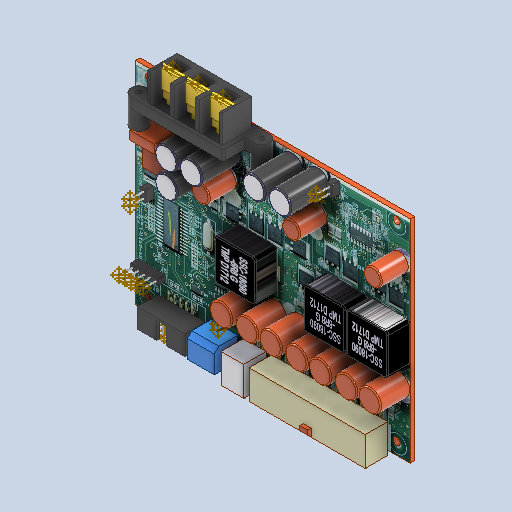
# Autodesk Inventor part: N40L
Saved by Autodesk Inventor 2022 (Build 260153000, 153)
## iProperties
Company: Hitatchi
Created: 2022-10-18
Checked By: Баранчук
Material: Phenolic Resin
Document SubType Name: Modeling
Density: 1.38 g/cm^3
Appearance: Smooth - Light Orange
Categories: <MemberInstance><Categories><Category DisplayName="" Mnemonic="CABLEANDHARNESS" InternalName="e4a7e005-5e42-4d16-b293-125e7f0d0512"><Category DisplayName="" Mnemonic="CONNECTORS" InternalName="6f634eba-a678-4820-a31d-2c2d5ee6728e"><CategoryParameter DisplayName="" Mnemonic="REFDES" InternalName="c3740e8c-60ab-4d5d-8584-52b73222f2f0"/><Category DisplayName="" Mnemonic="DISCRETEWIRE" InternalName="9a3407de-09b2-4cdb-8c40-9708d5144a28"/></Category></Category></Categories><FamilyTemplate><FamilyTemplateParameters></FamilyTemplateParameters></FamilyTemplate><CategoryParameterMap><ParamToTemplateMap><ParamToTemplate CategoryParameter="//CategoryParameter[@InternalName='c3740e8c-60ab-4d5d-8584-52b73222f2f0']" ConstantValue=""/></ParamToTemplateMap></CategoryParameterMap></MemberInstance>
Catalog Web Link: https://www.dont.ru/mini-box-M4-ATX-avtomobilnyj-6-30V-250W.id13127.html
Mass: 87.5567 g
Surface Area: 531.447 cm^2
Volume: 63.4469 cm^3
Part Number: N40L
Description: M4 ATX 250W AC-DC Powersupply
GlobalPropertyList: <PropertyList/>
Title: M4-ATX (6-30V) 250W AC-DC Powersupplu
Author: Tezeuz
Autodesk Inventor part; units mm, degrees
ref_plane "YZ Plane" through (0, 0, 0) normal (1, 0, 0) x (0, 1, 0)
ref_plane "XZ Plane" through (0, 0, 0) normal (0, 1, 0) x (-1, 0, 0)
ref_plane "XY Plane" through (0, 0, 0) normal (0, 0, 1) x (1, 0, 0)
sketch "Sketch1" plane through (0, 0, 0) normal (0, 0, 1) x (1, 0, 0)
  line L0 (-61, 47) -> (61, 47)
  line L1 (61, 47) -> (61, -47)
  line L2 (61, -47) -> (-61, -47)
  line L3 (-61, -47) -> (-61, 47)
  line L4 (-55, 43.5) -> (55, 43.5) construction
  line L5 (55, 43.5) -> (55, -41.5) construction
  line L6 (55, -41.5) -> (-55, -41.5) construction
  line L7 (-55, -41.5) -> (-55, 43.5) construction
  point P0 (0, 0)
  point P1 (61, 0)
  point P2 (0, 47)
  dimension "d0" = 122
  dimension "d1" = 94
  dimension "d4" = 85
  dimension "d5" = 110
  dimension "d6" = 3.5
  dimension "d7" = 6
  dimension "d8" = 5.5
  constraints: 16 end point, 4 parallel, 2 horizontal, 2 midpoint, 2 perpendicular, 1 horizontal alignment, 1 vertical alignment
  measures "d0" distance of L0.start L0.end
  measures "d1" distance of L0.end L1.end
  measures "d4" distance of L4.end L5.end
  measures "d5" distance of L4.start L4.end
  measures "d6" distance between parallel lines of L0 L4
  measures "d7" distance between parallel lines of L1 L5
  measures "d8" distance between parallel lines of L2 L6
extrude "Extrusion1" add sketch "Sketch1" against normal blind 2
hole "Hole1" at (-55, 43.5, 0) at (55, 43.5, 0) at (55, -41.5, 0) at (-55, -41.5, 0) direction (0, 0, -1) diameter 3.2 depth 2
sketch "Sketch3" plane through (0, 0, 0) normal (0, 0, 1) x (1, 0, 0)
  line L0 (-0.5, -36) -> (51, -36)
  line L1 (51, -36) -> (51, -49)
  line L2 (51, -49) -> (-0.5, -49)
  line L3 (-0.5, -49) -> (-0.5, -36)
  line L4 (-61, -47) -> (61, -47) projected
  line L5 (61, -47) -> (61, 47) projected
  line L6 (-13, -36) -> (-3, -36)
  line L7 (-3, -36) -> (-3, -49)
  line L8 (-3, -49) -> (-13, -49)
  line L9 (-13, -49) -> (-13, -36)
  line L10 (-27.5, -36) -> (-15.5, -36)
  line L11 (-15.5, -36) -> (-15.5, -46)
  line L12 (-15.5, -46) -> (-27.5, -46)
  line L13 (-27.5, -46) -> (-27.5, -36)
  line L14 (-51, -38.2) -> (-30, -38.2)
  line L15 (-30, -38.2) -> (-30, -47.2)
  line L16 (-30, -47.2) -> (-51, -47.2)
  line L17 (-51, -47.2) -> (-51, -38.2)
  point P0 (0, 0)
  point P1 (25.25, -36)
  point P2 (-51, -47)
  point P3 (-30, -47)
  dimension "d22" = 2
  dimension "d23" = 13
  dimension "d24" = 51.5
  dimension "d67" = 10
  dimension "d68" = 10
  dimension "d69" = 2.5
  dimension "d70" = 12
  dimension "d71" = 10
  dimension "d72" = 2.5
  dimension "d73" = 2.5
  dimension "d74" = 1
  dimension "d75" = 21
  dimension "d76" = 9
  dimension "d77" = 0.2
  constraints: 32 end point, 8 parallel, 4 horizontal, 4 perpendicular, 2 collinear, 1 midpoint
  measures "d22" distance between parallel lines of L4 L2
  measures "d23" distance of L0.end L1.end
  measures "d24" distance of L0.start L0.end
  measures "d67" distance between parallel lines of L5 L1
  measures "d68" distance of L7.end L8.end
  measures "d69" distance between parallel lines of L3 L7
  measures "d70" distance of L10.start L10.end
  measures "d71" distance of L10.end L11.end
  measures "d72" distance between parallel lines of L9 L11
  measures "d73" distance between parallel lines of L13 L15
  measures "d74" distance between parallel lines of L4 L12
  measures "d75" distance of L14.start L14.end
  measures "d76" distance of L16.end L14.start
  measures "d77" distance between parallel lines of L16 L4
extrude "Extrusion3" add sketch "Sketch3" along normal blind 10 separate body contours L0 L1 L4 L3 | L4 L1 L2 L3 | L9 L6 L7 L4 | L4 L7 L8 L9
sketch "Sketch4" plane through (0, 0, 0) normal (0, 0, 1) x (1, 0, 0)
  circle A0 centre (55.8, -19) radius 5
  line L0 (-61, -47) -> (61, -47) projected
  circle A1 centre (1.3, -19) radius 5
  circle A2 centre (11.8, -19) radius 5
  circle A3 centre (23.3, -19) radius 5
  circle A4 centre (33.8, -19) radius 5
  circle A5 centre (45.3, -19) radius 5
  circle A6 centre (-10.2, -19) radius 5
  line L1 (61, -47) -> (61, 47) projected
  line L2 (-10.2, -19) -> (1.3, -19) construction
  line L3 (1.3, -19) -> (11.8, -19) construction
  line L4 (11.8, -19) -> (23.3, -19) construction
  line L5 (23.3, -19) -> (33.8, -19) construction
  line L6 (33.8, -19) -> (45.3, -19) construction
  line L7 (45.3, -19) -> (55.8, -19) construction
  line L8 (-10.2, -19) -> (-15.2, -19) construction
  line L9 (55.8, -19) -> (61, -19) construction
  line L10 (61, 47) -> (61, -47) projected
  point P0 (0, 0)
  point P1 (51, -47)
  dimension "d28" = 28
  dimension "d48" = 10.5
  dimension "d49" = 11.5
  dimension "d50" = 10.5
  dimension "d51" = 11.5
  dimension "d52" = 10.5
  dimension "d53" = 11.5
  dimension "d54" = 10
  dimension "d55" = 5.2
  dimension "d110" = 76.2
  constraints: 16 end point, 6 centre point, 5 equal radius, 5 horizontal, 3 collinear, 1 horizontal alignment, 1 point on line, 3 other
  measures "d28" distance from line of L0 L7.end
  measures "d48" distance of L7.end L6.end
  measures "d49" distance of L6.end L5.end
  measures "d50" distance of L5.end L4.end
  measures "d51" distance of L4.end L3.end
  measures "d52" distance of L3.end L2.end
  measures "d53" distance of L2.end L2.start
  measures "d54" diameter of A0
  measures "d55" distance from line of L1 L7.end
  measures "d110" distance of L8.end L9.end
extrude "Extrusion4" add sketch "Sketch4" along normal blind 13 bodies 1
sketch "Sketch5" plane through (0, 0, 0) normal (0, 0, 1) x (1, 0, 0)
  circle A0 centre (8.5, 41.2) radius 5
  circle A1 centre (20, 41.2) radius 5
  circle A2 centre (-19.5, 33) radius 5
  circle A3 centre (-30.5, 33) radius 5
  circle A4 centre (-30.5, 22) radius 5
  line L0 (-30.5, 33) -> (-19.5, 33) construction
  line L1 (8.5, 41.2) -> (20, 41.2) construction
  line L2 (3.5, 41.2) -> (25, 41.2) construction
  line L3 (61, -47) -> (61, 47) projected
  line L4 (20, 41.2) -> (20, 46.2) construction
  line L5 (61, 47) -> (-61, 47) projected
  circle A5 centre (56.2, 28.2) radius 4
  circle A6 centre (19.9, 28.2) radius 4
  circle A7 centre (-20.2659, 22) radius 4
  line L6 (19.9, 28.2) -> (56.2, 28.2) construction
  line L7 (56.2, 28.2) -> (61, 28.2) construction
  line L8 (56.2, 28.2) -> (56.2, 32.2) construction
  line L9 (19.9, 28.2) -> (15.9, 28.2) construction
  line L10 (-30.5, 33) -> (-30.5, 38) construction
  line L11 (-30.5, 33) -> (-35.5, 33) construction
  line L12 (-30.5, 22) -> (-30.5, 17) construction
  line L13 (-19.5, 33) -> (-14.5, 33) construction
  line L14 (-30.5, 22) -> (-20.2659, 22) construction
  line L15 (-61, -47) -> (61, -47) projected
  line L16 (-20.2659, 22) -> (-20.2659, 18) construction
  line L17 (-19.5, 33) -> (-19.5, 38) construction
  line L18 (-61, 47) -> (-61, -47) projected
  point P0 (0, 0)
  point P1 (-25, 62)
  point P2 (-25, 33)
  point P3 (1, 47)
  point P4 (60.2, 28.2)
  dimension "d38" = 10
  dimension "d43" = 10
  dimension "d39" = 10
  dimension "d41" = 10
  dimension "d42" = 10
  dimension "d132" = 21.5
  dimension "d133" = 36
  dimension "d134" = 0.8
  dimension "d135" = 8
  dimension "d136" = 14.8
  dimension "d137" = 0.8
  dimension "d138" = 44.3
  dimension "d139" = 21
  dimension "d140" = 21
  dimension "d141" = 64
  dimension "d144" = 30.5
  constraints: 30 end point, 8 point on circle, 6 horizontal, 5 point on line, 4 centre point, 4 vertical, 4 vertical alignment, 2 horizontal alignment, 2 perpendicular, 1 coincident, 1 midpoint, 9 other
  measures "d39" diameter of A1
  measures "d41" diameter of A2
  measures "d42" diameter of A3
  measures "d132" distance of L2.end L2.start
  measures "d133" distance from line of L2.end L3
  measures "d134" distance from line of L5 L4.end
  measures "d135" diameter of A5
  measures "d136" distance from line of L5 L8.end
  measures "d137" distance from line of L3 A5.start
  measures "d138" distance of A5.start L9.end
  measures "d139" distance of L12.end L10.end
  measures "d140" distance of L13.end L11.end
  measures "d141" distance from line of L15 L12.end
  measures "d144" distance from line of L18 L12.end
extrude "Extrusion5" add sketch "Sketch5" along normal blind 17 separate body contours A0 | A1 | A2 | A3 | A4
sketch "Эскиз6" plane through (0, 0, 0) normal (0, 0, 1) x (1, 0, 0)
  line L0 (23.1, 8) -> (41.5, 8)
  line L1 (41.5, 8) -> (41.5, -10.4)
  line L2 (41.5, -10.4) -> (23.1, -10.4)
  line L3 (23.1, -10.4) -> (23.1, 8)
  line L4 (42.1, 8) -> (60.5, 8)
  line L5 (60.5, 8) -> (60.5, -10.4)
  line L6 (60.5, -10.4) -> (42.1, -10.4)
  line L7 (42.1, -10.4) -> (42.1, 8)
  line L8 (-16.6, 6.9) -> (1.8, 6.9)
  line L9 (1.8, 6.9) -> (1.8, -11.5)
  line L10 (1.8, -11.5) -> (-16.6, -11.5)
  line L11 (-16.6, -11.5) -> (-16.6, 6.9)
  line L12 (61, -47) -> (61, 47) projected
  line L13 (61, 47) -> (-61, 47) projected
  circle A0 centre (-10.2, -19) radius 5 projected
  line L14 (-10.2, -19) -> (-10.2, -14)
  point P0 (0, 0)
  point P1 (19.3803, 47)
  dimension "d56" = 18.4
  dimension "d57" = 21.3
  dimension "d58" = 37.4
  dimension "d59" = 0.5
  dimension "d60" = 39
  dimension "d61" = 2.5
  constraints: 26 end point, 6 parallel, 4 equal length, 3 horizontal, 3 perpendicular, 2 point on line, 1 vertical, 1 vertical alignment, 1 other
  measures "d56" distance of L10.end L8.start
  measures "d57" distance between parallel lines of L3 L9
  measures "d58" distance between parallel lines of L5 L3
  measures "d59" distance between parallel lines of L12 L5
  measures "d60" distance between parallel lines of L4 L13
extrude "Выдавливание6" add sketch "Эскиз6" along normal blind 9.5 separate body contours L0 L1 L2 L3 | L4 L5 L6 L7 | L8 L9 L10 L11
fillet "Сопряжение2" radius 1.5 12 edges at (-16.6, -11.5, 4.75) (1.8, -11.5, 4.75) (-16.6, 6.9, 4.75) (1.8, 6.9, 4.75) (23.1, -10.4, 4.75) (41.5, -10.4, 4.75) (42.1, -10.4, 4.75) (60.5, -10.4, 4.75) (60.5, 8, 4.75) (41.5, 8, 4.75) (42.1, 8, 4.75) (23.1, 8, 4.75)
extrude "Выдавливание7" add sketch "Sketch3" along normal blind 10.5 separate body contours L10 L11 L12 L13
extrude "Выдавливание8" add sketch "Sketch3" along normal blind 9 separate body contours L17 L14 L15 L4
sketch "Эскиз7" plane through (0, 0, 10) normal (0, 0, 1) x (1, 0, 0)
  line L0 (-0.5, -49) -> (51, -49) projected
  line L1 (23.5, -45.5) -> (27, -45.5)
  line L2 (27, -45.5) -> (27, -49)
  line L3 (27, -49) -> (23.5, -49)
  line L4 (23.5, -49) -> (23.5, -45.5)
  point P0 (0, 0)
  point P1 (25.25, -49)
  point P2 (25.25, -49)
  dimension "d82" = 3.5
  constraints: 8 end point, 3 midpoint, 2 parallel, 2 perpendicular, 1 horizontal
  measures "d82" distance of L1.start L1.end
extrude "Выдавливание9" add sketch "Эскиз7" along normal blind 1.5 bodies 2
chamfer "Фаска1" distance 1.5 angle 45 1 edges at (25.25, -49, 11.5)
sketch "Эскиз8" plane through (0, 0, 0) normal (0, 0, 1) x (1, 0, 0)
  line L0 (-60.2, -28.9) -> (-47.7, -28.9)
  line L1 (-47.7, -28.9) -> (-47.7, -31.5)
  line L2 (-47.7, -31.5) -> (-60.2, -31.5)
  line L3 (-60.2, -31.5) -> (-60.2, -28.9)
  line L4 (-55.7, 2.7) -> (-53.1, 2.7)
  line L5 (-53.1, 2.7) -> (-53.1, -2.5)
  line L6 (-53.1, -2.5) -> (-55.7, -2.5)
  line L7 (-55.7, -2.5) -> (-55.7, 2.7)
  line L8 (-54.4, 2.7) -> (-54.4, -2.5) construction
  circle A0 centre (-54.4, 1.4) radius 0.35
  circle A1 centre (-54.4, -1.2) radius 0.35
  line L9 (-54.4, 1.4) -> (-54.4, -1.2) construction
  line L10 (-60.2, -30.2) -> (-47.7, -30.2) construction
  circle A2 centre (-53.95, -30.2) radius 0.35
  circle A3 centre (-51.35, -30.2) radius 0.35
  circle A4 centre (-48.75, -30.2) radius 0.35
  circle A5 centre (-56.55, -30.2) radius 0.35
  circle A6 centre (-59.15, -30.2) radius 0.35
  line L11 (-61, 47) -> (-61, -47) projected
  line L12 (-61, -47) -> (61, -47) projected
  line L13 (26.9, 45.8) -> (29.5, 45.8)
  line L14 (29.5, 45.8) -> (29.5, 40.6)
  line L15 (29.5, 40.6) -> (26.9, 40.6)
  line L16 (26.9, 40.6) -> (26.9, 45.8)
  line L17 (28.2, 45.8) -> (28.2, 40.6) construction
  circle A7 centre (28.2, 44.5) radius 0.35
  circle A8 centre (28.2, 41.9) radius 0.35
  line L18 (28.2, 44.5) -> (28.2, 41.9) construction
  line L19 (-16.6, -25.8) -> (-14, -25.8)
  line L20 (-14, -25.8) -> (-14, -31)
  line L21 (-14, -31) -> (-16.6, -31)
  line L22 (-16.6, -31) -> (-16.6, -25.8)
  line L23 (-15.3, -25.8) -> (-15.3, -31) construction
  circle A9 centre (-15.3, -27.1) radius 0.35
  circle A10 centre (-15.3, -29.7) radius 0.35
  line L24 (-15.3, -27.1) -> (-15.3, -29.7) construction
  line L25 (61, 47) -> (-61, 47) projected
  line L26 (61, -47) -> (61, 47) projected
  point P0 (0, 0)
  point P1 (-54.4, 0.1)
  point P2 (28.2, 43.2)
  point P3 (-15.3, -28.4)
  point P4 (19.3803, 47)
  dimension "d88" = 2.6
  dimension "d89" = 0.7
  dimension "d90" = 2.6
  dimension "d91" = 12.5
  dimension "d92" = 2.6
  dimension "d93" = 2.6
  dimension "d94" = 2.6
  dimension "d95" = 0.8
  dimension "d96" = 15.5
  dimension "d97" = 5.3
  dimension "d98" = 44.5
  dimension "d100" = 1.3
  dimension "d101" = 2.6
  dimension "d102" = 1.3
  dimension "d103" = 2.6
  dimension "d104" = 1.3
  dimension "d105" = 2.6
  dimension "d106" = 1.2
  dimension "d107" = 31.5
  dimension "d108" = 16
  dimension "d111" = 75
  constraints: 46 end point, 15 midpoint, 11 centre point, 10 equal radius, 10 point on line, 8 parallel, 4 horizontal, 4 perpendicular, 3 collinear, 3 equal length
  measures "d88" distance of A3.centre A2.centre
  measures "d89" diameter of A2
  measures "d90" distance of L2.end L0.start
  measures "d91" distance of L0.start L0.end
  measures "d92" distance of A4.centre A3.centre
  measures "d93" distance of A2.centre A5.centre
  measures "d94" distance of A5.centre A6.centre
  measures "d95" distance between parallel lines of L3 L11
  measures "d96" distance between parallel lines of L12 L2
  measures "d97" distance between parallel lines of L7 L11
  measures "d98" distance between parallel lines of L6 L12
  measures "d100" distance from line of L6 L9.end
  measures "d101" distance of L9.end L9.start
  measures "d102" distance from line of L15 L18.end
  measures "d103" distance of L18.end L18.start
  measures "d104" distance from line of L21 L24.end
  measures "d105" distance of L24.end L24.start
  measures "d106" distance between parallel lines of L13 L25
  measures "d107" distance between parallel lines of L26 L14
  measures "d108" distance between parallel lines of L21 L12
  measures "d111" distance between parallel lines of L20 L26
extrude "Выдавливание10" add sketch "Эскиз8" along normal blind 3 separate body contours L0 L1 L2 L3 | L4 L5 L6 L7 | L13 L14 L15 L16 | L19 L20 L21 L22
extrude "Выдавливание11" add sketch "Эскиз8" along normal blind 9.5 separate body contours A0 | A1 | A2 | A3 | A4 | A5 | A6 | A7 | A8 | A9 | A10
fillet "Сопряжение4" radius 0.2 12 edges at (-55.7, -2.5, 1.5) (-53.1, -2.5, 1.5) (-55.7, 2.7, 1.5) (-60.2, -28.9, 1.5) (-60.2, -31.5, 1.5) (-47.7, -31.5, 1.5) (-47.7, -28.9, 1.5) (-53.1, 2.7, 1.5) (29.5, 40.6, 1.5) (29.5, 45.8, 1.5) (26.9, 40.6, 1.5) (26.9, 45.8, 1.5)
chamfer "Фаска2" distance 2 angle 45 1 edges at (-21.5, -36, 10.5)
sketch "Эскиз9" plane through (-0.5, -49, 0) normal (0, -1, 0) x (1, 0, 0)
  line L0 (-12.5, 0) -> (-2.5, 0) projected
  line L1 (-2.5, 0) -> (-2.5, 10) projected
  line L2 (-12.5, 10) -> (-2.5, 10) projected
  line L3 (-12.5, 0) -> (-12.5, 10) projected
  line L4 (24, 10) -> (27.5, 10) projected
  line L5 (0, 10) -> (24, 10) projected
  line L6 (0, 0) -> (0, 10) projected
  line L7 (0, 0) -> (51.5, 0) projected
  line L8 (51.5, 0) -> (51.5, 10) projected
  line L9 (27.5, 10) -> (51.5, 10) projected
  line L10 (-3.6, 8.9) -> (-3.6, 1.1)
  line L11 (-3.6, 1.1) -> (-11.4, 1.1)
  line L12 (-11.4, 1.1) -> (-11.4, 8.9)
  line L13 (-11.4, 8.9) -> (-3.6, 8.9)
  line L14 (24, 8.9) -> (27.5, 8.9)
  line L15 (27.5, 8.9) -> (50.4, 8.9)
  line L16 (50.4, 8.9) -> (50.4, 1.1)
  line L17 (50.4, 1.1) -> (1.1, 1.1)
  line L18 (1.1, 1.1) -> (1.1, 8.9)
  line L19 (1.1, 8.9) -> (24, 8.9)
  line L20 (-11.4, 8.9) -> (-7.75, 8.9)
  line L21 (-7.75, 8.9) -> (-7.75, 5.25)
  line L22 (-7.75, 5.25) -> (-11.4, 5.25)
  line L23 (-11.4, 5.25) -> (-11.4, 8.9)
  line L24 (-11.4, 8.9) -> (-7.75, 5.25) construction
  line L25 (-7.75, 8.9) -> (-11.4, 5.25) construction
  line L26 (-7.25, 8.9) -> (-3.6, 8.9)
  line L27 (-3.6, 8.9) -> (-3.6, 5.25)
  line L28 (-3.6, 5.25) -> (-7.25, 5.25)
  line L29 (-7.25, 5.25) -> (-7.25, 8.9)
  line L30 (-7.25, 8.9) -> (-3.6, 5.25) construction
  line L31 (-3.6, 8.9) -> (-7.25, 5.25) construction
  line L32 (-11.4, 4.75) -> (-7.75, 4.75)
  line L33 (-7.75, 4.75) -> (-7.75, 1.1)
  line L34 (-7.75, 1.1) -> (-11.4, 1.1)
  line L35 (-11.4, 1.1) -> (-11.4, 4.75)
  line L36 (-11.4, 4.75) -> (-7.75, 1.1) construction
  line L37 (-7.75, 4.75) -> (-11.4, 1.1) construction
  line L38 (-7.25, 4.75) -> (-3.6, 4.75)
  line L39 (-3.6, 4.75) -> (-3.6, 1.1)
  line L40 (-3.6, 1.1) -> (-7.25, 1.1)
  line L41 (-7.25, 1.1) -> (-7.25, 4.75)
  line L42 (-7.25, 4.75) -> (-3.6, 1.1) construction
  line L43 (-3.6, 4.75) -> (-7.25, 1.1) construction
  circle A0 centre (-9.575, 7.075) radius 0.5
  circle A1 centre (-5.425, 7.075) radius 0.5
  circle A2 centre (-9.575, 2.925) radius 0.5
  circle A3 centre (-5.425, 2.925) radius 0.5
  line L44 (4.75, 1.1) -> (1.1, 1.1)
  line L45 (1.1, 1.1) -> (1.1, 4.75)
  line L46 (1.1, 4.75) -> (4.75, 4.75)
  line L47 (4.75, 4.75) -> (4.75, 1.1)
  line L48 (4.75, 1.1) -> (1.1, 4.75) construction
  line L49 (1.1, 1.1) -> (4.75, 4.75) construction
  line L50 (4.75, 8.9) -> (1.1, 8.9)
  line L51 (1.1, 8.9) -> (1.1, 5.25)
  line L52 (1.1, 5.25) -> (4.75, 5.25)
  line L53 (4.75, 5.25) -> (4.75, 8.9)
  line L54 (4.75, 8.9) -> (1.1, 5.25) construction
  line L55 (1.1, 8.9) -> (4.75, 5.25) construction
  circle A4 centre (2.925, 2.925) radius 0.5
  circle A5 centre (2.925, 7.075) radius 0.5
  point P0 (0.5, 0)
  point P1 (-7.25, 8.9)
  point P2 (-7.25, 1.1)
  point P3 (-3.6, 4.75)
  point P4 (-7.75, 1.1)
  point P5 (-11.4, 5.25)
  point P6 (-7.75, 8.9)
  point P7 (4.75, 1.1)
  dimension "d120" = 1.1
  dimension "d121" = 1.1
  dimension "d122" = 0.5
  dimension "d123" = 0.5
  dimension "d124" = 1
  constraints: 92 end point, 12 midpoint, 12 parallel, 9 equal length, 6 centre point, 6 coincident, 6 horizontal, 6 perpendicular, 5 equal radius, 1 collinear, 8 other
  measures "d120" distance between parallel lines of L2 L13
  measures "d121" distance between parallel lines of L5 L19
  measures "d122" distance between parallel lines of L29 L21
  measures "d123" distance between parallel lines of L38 L28
  measures "d124" diameter of A1
extrude "Выдавливание12" cut sketch "Эскиз9" against normal blind 9.5 contours L10 L28 L29 L13 | L10 L11 L41 L38 | L21 L22 L12 L13 | L11 L12 L32 L33 bodies 2
extrude "Выдавливание13" cut sketch "Эскиз9" against normal blind 9.5 contours L53 L52 L18 L19 | L17 L18 L46 L47 bodies 2
pattern_linear "Прямоуг.массив1" count 12 spacing 4.15 along (1, 0, 0) of "Выдавливание13" bodies 2
extrude "Выдавливание14" add sketch "Sketch5" along normal blind 12 contours A5 | A6 | A7 bodies 1
fillet "Сопряжение3" radius 0.5 15 edges at (-15.2, -19, 13) (-3.7, -19, 13) (6.8, -19, 13) (18.3, -19, 13) (28.8, -19, 13) (40.3, -19, 13) (50.8, -19, 13) (-24.2659, 22, 12) (15.9, 28.2, 12) (52.2, 28.2, 12) (15, 41.2, 17) (3.5, 41.2, 17) (-24.5, 33, 17) (-35.5, 33, 17) (-35.5, 22, 17)
sketch "Эскиз10" plane through (-61, 47, 0) normal (0, 1, 0) x (1, 0, 0)
  line L0 (0, 0) -> (0, 2) construction
  line L1 (55.5, -16.5) -> (18.5, -16.5)
  line L2 (18.5, -16.5) -> (18.5, 0)
  line L3 (18.5, 0) -> (55.5, 0)
  line L4 (55.5, 0) -> (55.5, -16.5)
  line L5 (55.5, -16.5) -> (18.5, 0) construction
  line L6 (18.5, -16.5) -> (55.5, 0) construction
  line L7 (51.5, -3.5) -> (59.5, -3.5) construction
  line L8 (51.5, -7) -> (59.5, -7)
  line L9 (59.5, 0) -> (51.5, 0)
  arc A0 (51.5, 0) -> (51.5, -7) centre (51.5, -3.5) ccw
  arc A1 (59.5, -7) -> (59.5, 0) centre (59.5, -3.5) ccw
  line L10 (22.5, -13) -> (14.5, -13) construction
  line L11 (22.5, -9.5) -> (14.5, -9.5)
  line L12 (14.5, -16.5) -> (22.5, -16.5)
  arc A2 (22.5, -16.5) -> (22.5, -9.5) centre (22.5, -13) ccw
  arc A3 (14.5, -9.5) -> (14.5, -16.5) centre (14.5, -13) ccw
  line L13 (59.5, -3.5) -> (63, -3.5) construction
  line L14 (14.5, -13) -> (11, -13) construction
  circle A4 centre (59.5, -3.5) radius 1.15
  circle A5 centre (14.5, -13) radius 1.15
  circle A6 centre (59.5, -3.5) radius 3.5
  circle A7 centre (14.5, -13) radius 3.5
  line L15 (122, 0) -> (0, 0) projected
  point P0 (61, 0)
  point P1 (37, -8.25)
  point P2 (55.5, -3.5)
  point P3 (18.5, -13)
  point P4 (18.5, -9.5)
  point P5 (18.5, -16.5)
  point P6 (55.5, -7)
  dimension "d149" = 37
  dimension "d151" = 52
  dimension "d152" = 16.5
  dimension "d154" = 7
  dimension "d155" = 2.3
  dimension "d156" = 11
  constraints: 32 end point, 10 point on circle, 8 tangent, 7 centre point, 5 parallel, 4 coincident, 4 midpoint, 3 collinear, 3 equal radius, 3 perpendicular, 2 horizontal, 2 point on line, 3 other
  measures "d149" distance between parallel lines of L2 L4
  measures "d151" horizontal distance of L13.end L14.end
  measures "d152" distance of L1.end L2.end
  measures "d154" distance between parallel lines of L11 L12
  measures "d155" diameter of A5
  measures "d156" distance from line of L0 L14.end
extrude "Выдавливание15" add sketch "Эскиз10" against normal blind 3 separate body
extrude "Выдавливание16" add sketch "Эскиз10" against normal blind 11 contours A6 A1 | A3 A7 bodies 9
move faces "Перенос1" translate (0, 1.5, 0) faces at (-30.1667, 47, 5.5)
fillet "Сопряжение5" radius 1 4 edges at (-5.5, 47.75, 16.5) (-5.5, 45.5, 16.5) (-42.5, 47.75, 0) (-42.5, 45.5, 0)
sketch "Эскиз11" plane through (-61, 47, 0) normal (0, 1, 0) x (1, 0, 0)
  line L0 (53.5, -15) -> (20.5, -15)
  line L1 (20.5, -15) -> (20.5, -2)
  line L2 (20.5, -2) -> (53.5, -2)
  line L3 (53.5, -2) -> (53.5, -15)
  line L4 (14.5, -16.5) -> (54.5, -16.5) projected
  line L5 (55.5, -15.5) -> (55.5, -7) projected
  line L6 (32.5, -15) -> (41.5, -15)
  line L7 (41.5, -15) -> (41.5, -9.7)
  line L8 (41.5, -9.7) -> (32.5, -9.7)
  line L9 (32.5, -9.7) -> (32.5, -15)
  line L10 (42, -9.7) -> (32, -9.7)
  line L11 (32, -9.7) -> (32, -8.5)
  line L12 (32, -8.5) -> (42, -8.5)
  line L13 (42, -8.5) -> (42, -9.7)
  line L14 (40.25, -8.5) -> (33.75, -8.5)
  line L15 (33.75, -8.5) -> (33.75, -4.5)
  line L16 (33.75, -4.5) -> (40.25, -4.5)
  line L17 (40.25, -4.5) -> (40.25, -8.5)
  point P0 (61, 0)
  point P1 (37, -8.5)
  point P2 (37, -15)
  point P3 (37, -9.7)
  dimension "d162" = 33
  dimension "d163" = 13
  dimension "d164" = 1.5
  dimension "d165" = 2
  dimension "d166" = 9
  dimension "d167" = 10
  dimension "d168" = 6.5
  dimension "d169" = 2.5
  dimension "d170" = 1.2
  dimension "d171" = 4
  constraints: 32 end point, 8 parallel, 6 midpoint, 4 horizontal, 4 perpendicular, 1 point on line
  measures "d162" distance of L0.start L0.end
  measures "d163" distance of L0.end L1.end
  measures "d164" distance between parallel lines of L4 L0
  measures "d165" distance between parallel lines of L5 L3
  measures "d166" distance between parallel lines of L9 L7
  measures "d167" distance of L10.start L10.end
  measures "d168" distance between parallel lines of L15 L17
  measures "d169" distance between parallel lines of L2 L16
  measures "d170" distance of L10.end L11.end
  measures "d171" distance of L14.end L15.end
extrude "Выдавливание17" add sketch "Эскиз11" along normal blind 14 bodies 9
extrude "Выдавливание18" cut sketch "Эскиз11" along normal blind 14 contours L0 L9 L8 L7 | L8 L10 L11 L12 L13 | L12 L15 L16 L17 bodies 9
pattern_linear "Прямоуг.массив2" count 3 spacing 11 along (-1, 0, 0) of "Выдавливание18" first direction both ways yes bodies 9
sketch "Эскиз12" plane through (-61, 61, 0) normal (0, 1, 0) x (1, 0, 0)
  line L0 (42, -9.7) -> (42, -8.5) projected
  line L1 (32, -9.7) -> (32, -8.5) projected
  line L2 (42, -9.7) -> (32, -9.7)
  line L3 (32, -9.7) -> (32, -8.5)
  line L4 (32, -8.5) -> (42, -8.5)
  line L5 (42, -8.5) -> (42, -9.7)
  line L6 (45.5, -8.5) -> (33.5, -8.5) projected
  line L7 (39.5, -9.7) -> (34.5, -9.7)
  line L8 (34.5, -9.7) -> (34.5, -8.5)
  line L9 (34.5, -8.5) -> (39.5, -8.5)
  line L10 (39.5, -8.5) -> (39.5, -9.7)
  point P0 (61, 0)
  point P1 (37, -9.7)
  dimension "d179" = 5
  constraints: 16 end point, 4 parallel, 2 horizontal, 2 midpoint, 2 perpendicular, 2 point on line
  measures "d179" distance between parallel lines of L8 L10
extrude "Выдавливание19" add sketch "Эскиз12" against normal blind 12.5 separate body
extrude "Выдавливание20" add sketch "Эскиз12" against normal blind 21.5 contours L2 L8 L4 L10 bodies 10
sketch "Эскиз13" plane through (-29, 61, 9.7) normal (0, 0, 1) x (1, 0, 0)
  line L0 (9, -8.5) -> (1, -8.5)
  line L1 (1, -8.5) -> (1, -0.5)
  line L2 (1, -0.5) -> (9, -0.5)
  line L3 (9, -0.5) -> (9, -8.5)
  line L4 (9, -8.5) -> (1, -0.5) construction
  line L5 (1, -8.5) -> (9, -0.5) construction
  line L6 (21.5, 0) -> (-11.5, 0) projected
  line L7 (5, 0) -> (5, -0.5)
  line L8 (0.5, -12.5) -> (0.5, 0) projected
  point P0 (29, -61)
  point P1 (5, -4.5)
  point P2 (5, -0.25)
  point P3 (0.5, -14)
  dimension "d184" = 0.5
  dimension "d185" = 0.5
  constraints: 14 end point, 5 midpoint, 2 parallel, 2 perpendicular, 1 horizontal, 1 vertical
  measures "d184" distance between parallel lines of L6 L2
  measures "d185" distance between parallel lines of L8 L1
extrude "Выдавливание21" add sketch "Эскиз13" along normal blind 1 bodies 10
pattern_linear "Прямоуг.массив3" count 3 spacing 11 along (-1, 0, 0) first direction both ways yes bodies 10
sketch "Эскиз14" plane through (0, 0, 0) normal (0, 0, 1) x (1, 0, 0)
  line L0 (-48.5, 34) -> (-37.5, 34)
  line L1 (-37.5, 34) -> (-37.5, 30)
  line L2 (-37.5, 30) -> (-48.5, 30)
  line L3 (-48.5, 30) -> (-48.5, 34)
  line L4 (-49.5, 29) -> (-36.5, 29)
  line L5 (-36.5, 29) -> (-36.5, 16)
  line L6 (-36.5, 16) -> (-49.5, 16)
  line L7 (-49.5, 16) -> (-49.5, 29)
  line L8 (-43, 30) -> (-43, 29)
  line L9 (-61, 47) -> (-61, -47) projected
  line L10 (-61, -47) -> (61, -47) projected
  line L11 (61, 47) -> (-61, 47) projected
  point P0 (0, 0)
  dimension "d191" = 13
  dimension "d192" = 11
  dimension "d193" = 4
  dimension "d194" = 1
  dimension "d195" = 11.5
  dimension "d205" = 13
  constraints: 18 end point, 4 parallel, 3 perpendicular, 2 horizontal, 2 midpoint, 1 vertical
  measures "d191" distance of L5.end L6.end
  measures "d192" distance of L0.start L0.end
  measures "d193" distance between parallel lines of L2 L0
  measures "d194" distance between parallel lines of L4 L2
  measures "d195" distance between parallel lines of L7 L9
  measures "d205" distance between parallel lines of L0 L11
extrude "Выдавливание22" add sketch "Эскиз14" along normal blind 9 separate body contours L4 L5 L6 L7
extrude "Выдавливание23" add sketch "Эскиз14" along normal blind 15 separate body contours L0 L1 L2 L3
fillet "Сопряжение6" radius 1 4 edges at (-49.5, 29, 4.5) (-49.5, 16, 4.5) (-36.5, 16, 4.5) (-36.5, 29, 4.5)
fillet "Сопряжение7" radius 0.5 8 edges at (-49.2071, 16.2929, 9) (-43, 16, 9) (-36.7929, 16.2929, 9) (-36.5, 22.5, 9) (-36.7929, 28.7071, 9) (-43, 29, 9) (-49.2071, 28.7071, 9) (-49.5, 22.5, 9)
fillet "Сопряжение8" radius 0.5 24 edges at (-16.1607, 6.4607, 9.5) (-16.6, -2.3, 9.5) (-16.1607, -11.0607, 9.5) (-7.4, -11.5, 9.5) (1.3607, -11.0607, 9.5) (1.8, -2.3, 9.5) (1.3607, 6.4607, 9.5) (-7.4, 6.9, 9.5) (23.5393, 7.5607, 9.5) (23.1, -1.2, 9.5) (23.5393, -9.9607, 9.5) (32.3, -10.4, 9.5) (41.0607, -9.9607, 9.5) (41.5, -1.2, 9.5) (41.0607, 7.5607, 9.5) (32.3, 8, 9.5) (42.5393, 7.5607, 9.5) (42.1, -1.2, 9.5) (42.5393, -9.9607, 9.5) (51.3, -10.4, 9.5) (60.0607, -9.9607, 9.5) (60.5, -1.2, 9.5) (60.0607, 7.5607, 9.5) (51.3, 8, 9.5)
sketch "Эскиз15" plane through (-51, -47, 0) normal (0, -1, 0) x (1, 0, 0)
  line L0 (1.4, 7.6) -> (19.6, 7.6)
  line L1 (19.6, 7.6) -> (19.6, 1.4)
  line L2 (19.6, 1.4) -> (1.4, 1.4)
  line L3 (1.4, 1.4) -> (1.4, 7.6)
  line L4 (0, 9) -> (21, 9) projected
  line L5 (8.4, 9) -> (12.6, 9)
  line L6 (12.6, 9) -> (12.6, 7.6)
  line L7 (12.6, 7.6) -> (8.4, 7.6)
  line L8 (8.4, 7.6) -> (8.4, 9)
  line L9 (21, 0) -> (21, 9) projected
  line L10 (0, 0) -> (0, 9) projected
  line L11 (-10, 0) -> (112, 0) projected
  line L12 (5.5, 5.75) -> (8, 5.75) construction
  line L13 (8, 5.75) -> (8, 3.25) construction
  line L14 (8, 3.25) -> (5.5, 3.25) construction
  line L15 (5.5, 3.25) -> (5.5, 5.75) construction
  line L16 (8, 3.25) -> (10.5, 3.25) construction
  line L17 (10.5, 3.25) -> (10.5, 5.75) construction
  line L18 (10.5, 5.75) -> (8, 5.75) construction
  line L19 (8, 5.75) -> (8, 3.25) construction
  line L20 (10.5, 5.75) -> (13, 5.75) construction
  line L21 (13, 5.75) -> (13, 3.25) construction
  line L22 (13, 3.25) -> (10.5, 3.25) construction
  line L23 (10.5, 3.25) -> (10.5, 5.75) construction
  line L24 (13, 3.25) -> (15.5, 3.25) construction
  line L25 (15.5, 3.25) -> (15.5, 5.75) construction
  line L26 (15.5, 5.75) -> (13, 5.75) construction
  line L27 (13, 5.75) -> (13, 3.25) construction
  circle A0 centre (5.5, 5.75) radius 0.4
  circle A1 centre (8, 5.75) radius 0.4
  circle A2 centre (10.5, 5.75) radius 0.4
  circle A3 centre (13, 5.75) radius 0.4
  circle A4 centre (15.5, 5.75) radius 0.4
  circle A5 centre (15.5, 3.25) radius 0.4
  circle A6 centre (13, 3.25) radius 0.4
  circle A7 centre (10.5, 3.25) radius 0.4
  circle A8 centre (8, 3.25) radius 0.4
  line L28 (10.5, 7.6) -> (10.5, 5.75) construction
  line L29 (10.5, 3.25) -> (10.5, 1.4) construction
  point P0 (51, 0)
  dimension "d209" = 1.4
  dimension "d210" = 1.4
  dimension "d211" = 1.4
  dimension "d212" = 1.4
  dimension "d213" = 4.2
  dimension "d214" = 0.8
  dimension "d215" = 2.5
  dimension "d216" = 2.5
  constraints: 52 end point, 12 parallel, 9 centre point, 9 coincident, 8 equal radius, 7 equal length, 6 horizontal, 6 perpendicular, 3 midpoint, 1 point on line, 1 vertical
  measures "d209" distance between parallel lines of L4 L0
  measures "d210" distance between parallel lines of L9 L1
  measures "d211" distance between parallel lines of L10 L3
  measures "d212" distance between parallel lines of L11 L2
  measures "d213" distance between parallel lines of L8 L6
  measures "d214" diameter of A5
  measures "d215" distance of L24.end L25.end
  measures "d216" distance of L25.end L26.end
extrude "Выдавливание24" cut sketch "Эскиз15" against normal blind 7.5 contours L0 L1 L2 L3 | L8 L4 L6 L0 bodies 6
sketch "Эскиз16" plane through (0, 0, 0) normal (0, 0, 1) x (1, 0, 0)
  line L0 (-61, -47) -> (61, -47) projected
  line L1 (-61, 47) -> (-61, -47) projected
  line L2 (61, 47) -> (-61, 47) projected
  line L3 (61, -47) -> (61, 47) projected
  line L4 (-72.459, 69.2423) -> (75.2758, 69.2423) construction
  line L5 (75.2758, 69.2423) -> (75.2758, -67.9894) construction
  line L6 (75.2758, -67.9894) -> (-72.459, -67.9894) construction
  line L7 (-72.459, -67.9894) -> (-72.459, 69.2423) construction
  point P0 (0, 0)
  constraints: 2 other
sketch "Эскиз17" plane through (0, 0, 9.5) normal (0, 0, 1) x (1, 0, 0)
  line L0 (-34.23, 45.1182) -> (78.4545, 45.1182) construction
  line L1 (78.4545, 45.1182) -> (78.4545, -42.5253) construction
  line L2 (78.4545, -42.5253) -> (-34.23, -42.5253) construction
  line L3 (-34.23, -42.5253) -> (-34.23, 45.1182) construction
  arc A0 (43.6, 7.5) -> (42.6, 6.5) centre (43.6, 6.5) ccw projected
  line L4 (42.6, -8.9) -> (42.6, 6.5) projected
  arc A1 (42.6, -8.9) -> (43.6, -9.9) centre (43.6, -8.9) ccw projected
  line L5 (59, -9.9) -> (43.6, -9.9) projected
  arc A2 (59, -9.9) -> (60, -8.9) centre (59, -8.9) ccw projected
  line L6 (60, 6.5) -> (60, -8.9) projected
  arc A3 (60, 6.5) -> (59, 7.5) centre (59, 6.5) ccw projected
  line L7 (43.6, 7.5) -> (59, 7.5) projected
  point P0 (0, 0)
  constraints: 2 other
decal "Маркировка2"
sketch "Эскиз18" plane through (0, 0, 9.5) normal (0, 0, 1) x (1, 0, 0)
  arc A0 (24.6, 7.5) -> (23.6, 6.5) centre (24.6, 6.5) ccw projected
  line L0 (23.6, -8.9) -> (23.6, 6.5) projected
  arc A1 (23.6, -8.9) -> (24.6, -9.9) centre (24.6, -8.9) ccw projected
  line L1 (40, -9.9) -> (24.6, -9.9) projected
  arc A2 (40, -9.9) -> (41, -8.9) centre (40, -8.9) ccw projected
  line L2 (41, 6.5) -> (41, -8.9) projected
  arc A3 (41, 6.5) -> (40, 7.5) centre (40, 6.5) ccw projected
  line L3 (24.6, 7.5) -> (40, 7.5) projected
  line L4 (-59.4062, 48.5244) -> (67.999, 48.5244) construction
  line L5 (67.999, 48.5244) -> (67.999, -47.0296) construction
  line L6 (67.999, -47.0296) -> (-59.4062, -47.0296) construction
  line L7 (-59.4062, -47.0296) -> (-59.4062, 48.5244) construction
  point P0 (0, 0)
  constraints: 2 other
decal "Маркировка3"
sketch "Эскиз19" plane through (0, 0, 9.5) normal (0, 0, 1) x (1, 0, 0)
  arc A0 (-15.1, 6.4) -> (-16.1, 5.4) centre (-15.1, 5.4) ccw projected
  line L0 (-16.1, -10) -> (-16.1, 5.4) projected
  arc A1 (-16.1, -10) -> (-15.1, -11) centre (-15.1, -10) ccw projected
  line L1 (0.3, -11) -> (-15.1, -11) projected
  arc A2 (0.3, -11) -> (1.3, -10) centre (0.3, -10) ccw projected
  line L2 (1.3, 5.4) -> (1.3, -10) projected
  arc A3 (1.3, 5.4) -> (0.3, 6.4) centre (0.3, 5.4) ccw projected
  line L3 (-15.1, 6.4) -> (0.3, 6.4) projected
  line L4 (-78.8067, 72.5543) -> (89.0926, 72.5543) construction
  line L5 (89.0926, 72.5543) -> (89.0926, -53.3702) construction
  line L6 (89.0926, -53.3702) -> (-78.8067, -53.3702) construction
  line L7 (-78.8067, -53.3702) -> (-78.8067, 72.5543) construction
  point P0 (0, 0)
  constraints: 2 other
decal "Маркировка4"
sketch "Эскиз21" plane through (0, 0, -2) normal (0, 0, -1) x (-1, 0, 0)
  line L0 (73.3216, -51.1221) -> (-79.2594, -51.1221) construction
  line L1 (-79.2594, -51.1221) -> (-79.2594, 63.3137) construction
  line L2 (-79.2594, 63.3137) -> (73.3216, 63.3137) construction
  line L3 (73.3216, 63.3137) -> (73.3216, -51.1221) construction
  circle A0 centre (-55, -41.5) radius 1.6 projected
  circle A1 centre (55, 43.5) radius 1.6 projected
  circle A2 centre (-55, 43.5) radius 1.6 projected
  circle A3 centre (55, -41.5) radius 1.6 projected
  line L4 (-61, -47) -> (61, -47) projected
  line L5 (61, -47) -> (61, 47) projected
  line L6 (61, 47) -> (-61, 47) projected
  line L7 (-61, 47) -> (-61, -47) projected
  point P0 (0, 0)
  constraints: 2 other
decal "Маркировка5"
sketch "Эскиз22" plane through (-10.075, -49, 7.075) normal (0, -1, 0) x (1, 0, 0)
  circle A0 centre (0, 0) radius 0.5 projected
sketch "Эскиз23" plane through (-5.925, -49, 7.075) normal (0, -1, 0) x (1, 0, 0)
  circle A0 centre (0, 0) radius 0.5 projected
sketch "Эскиз24" plane through (-10.075, -49, 2.925) normal (0, -1, 0) x (1, 0, 0)
  circle A0 centre (0, 0) radius 0.5 projected
sketch "Эскиз25" plane through (-5.925, -49, 2.925) normal (0, -1, 0) x (1, 0, 0)
  circle A0 centre (0, 0) radius 0.5 projected
sketch "Эскиз26" plane through (-45.5, -47, 5.75) normal (0, -1, 0) x (1, 0, 0)
  circle A0 centre (0, 0) radius 0.4 projected
sketch "Эскиз27" plane through (-43, -47, 5.75) normal (0, -1, 0) x (1, 0, 0)
  circle A0 centre (0, 0) radius 0.4 projected
sketch "Эскиз28" plane through (-40.5, -47, 5.75) normal (0, -1, 0) x (1, 0, 0)
  circle A0 centre (0, 0) radius 0.4 projected
sketch "Эскиз29" plane through (-38, -47, 5.75) normal (0, -1, 0) x (1, 0, 0)
  circle A0 centre (0, 0) radius 0.4 projected
sketch "Эскиз30" plane through (-35.5, -47, 5.75) normal (0, -1, 0) x (1, 0, 0)
  circle A0 centre (0, 0) radius 0.4 projected
sketch "Эскиз31" plane through (-35.5, -47, 3.25) normal (0, -1, 0) x (1, 0, 0)
  circle A0 centre (0, 0) radius 0.4 projected
sketch "Эскиз32" plane through (-38, -47, 3.25) normal (0, -1, 0) x (1, 0, 0)
  circle A0 centre (0, 0) radius 0.4 projected
sketch "Эскиз33" plane through (-40.5, -47, 3.25) normal (0, -1, 0) x (1, 0, 0)
  circle A0 centre (0, 0) radius 0.4 projected
sketch "Эскиз34" plane through (-43, -47, 3.25) normal (0, -1, 0) x (1, 0, 0)
  circle A0 centre (0, 0) radius 0.4 projected
sketch "Эскиз35" plane through (2.425, -49, 7.075) normal (0, -1, 0) x (1, 0, 0)
  circle A0 centre (0, 0) radius 0.5 projected
sketch "Эскиз36" plane through (6.575, -49, 7.075) normal (0, -1, 0) x (1, 0, 0)
  circle A0 centre (0, 0) radius 0.5 projected
sketch "Эскиз37" plane through (10.725, -49, 7.075) normal (0, -1, 0) x (1, 0, 0)
  circle A0 centre (0, 0) radius 0.5 projected
sketch "Эскиз38" plane through (14.875, -49, 7.075) normal (0, -1, 0) x (1, 0, 0)
  circle A0 centre (0, 0) radius 0.5 projected
sketch "Эскиз39" plane through (19.025, -49, 7.075) normal (0, -1, 0) x (1, 0, 0)
  circle A0 centre (0, 0) radius 0.5 projected
sketch "Эскиз40" plane through (23.175, -49, 7.075) normal (0, -1, 0) x (1, 0, 0)
  circle A0 centre (0, 0) radius 0.5 projected
sketch "Эскиз41" plane through (27.325, -49, 7.075) normal (0, -1, 0) x (1, 0, 0)
  circle A0 centre (0, 0) radius 0.5 projected
sketch "Эскиз42" plane through (31.475, -49, 7.075) normal (0, -1, 0) x (1, 0, 0)
  circle A0 centre (0, 0) radius 0.5 projected
sketch "Эскиз43" plane through (35.625, -49, 7.075) normal (0, -1, 0) x (1, 0, 0)
  circle A0 centre (0, 0) radius 0.5 projected
sketch "Эскиз44" plane through (39.775, -49, 7.075) normal (0, -1, 0) x (1, 0, 0)
  circle A0 centre (0, 0) radius 0.5 projected
sketch "Эскиз45" plane through (43.925, -49, 7.075) normal (0, -1, 0) x (1, 0, 0)
  circle A0 centre (0, 0) radius 0.5 projected
sketch "Эскиз46" plane through (48.075, -49, 7.075) normal (0, -1, 0) x (1, 0, 0)
  circle A0 centre (0, 0) radius 0.5 projected
sketch "Эскиз47" plane through (48.075, -49, 2.925) normal (0, -1, 0) x (1, 0, 0)
  circle A0 centre (0, 0) radius 0.5 projected
sketch "Эскиз48" plane through (43.925, -49, 2.925) normal (0, -1, 0) x (1, 0, 0)
  circle A0 centre (0, 0) radius 0.5 projected
sketch "Эскиз49" plane through (39.775, -49, 2.925) normal (0, -1, 0) x (1, 0, 0)
  circle A0 centre (0, 0) radius 0.5 projected
sketch "Эскиз50" plane through (35.625, -49, 2.925) normal (0, -1, 0) x (1, 0, 0)
  circle A0 centre (0, 0) radius 0.5 projected
sketch "Эскиз51" plane through (31.475, -49, 2.925) normal (0, -1, 0) x (1, 0, 0)
  circle A0 centre (0, 0) radius 0.5 projected
sketch "Эскиз52" plane through (27.325, -49, 2.925) normal (0, -1, 0) x (1, 0, 0)
  circle A0 centre (0, 0) radius 0.5 projected
sketch "Эскиз53" plane through (23.175, -49, 2.925) normal (0, -1, 0) x (1, 0, 0)
  circle A0 centre (0, 0) radius 0.5 projected
sketch "Эскиз54" plane through (19.025, -49, 2.925) normal (0, -1, 0) x (1, 0, 0)
  circle A0 centre (0, 0) radius 0.5 projected
sketch "Эскиз55" plane through (14.875, -49, 2.925) normal (0, -1, 0) x (1, 0, 0)
  circle A0 centre (0, 0) radius 0.5 projected
sketch "Эскиз56" plane through (10.725, -49, 2.925) normal (0, -1, 0) x (1, 0, 0)
  circle A0 centre (0, 0) radius 0.5 projected
sketch "Эскиз57" plane through (6.575, -49, 2.925) normal (0, -1, 0) x (1, 0, 0)
  circle A0 centre (0, 0) radius 0.5 projected
sketch "Эскиз58" plane through (2.425, -49, 2.925) normal (0, -1, 0) x (1, 0, 0)
  circle A0 centre (0, 0) radius 0.5 projected
sketch "Эскиз59" plane through (-59.15, -30.2, 9.5) normal (0, 0, 1) x (1, 0, 0)
  circle A0 centre (0, 0) radius 0.35 projected
sketch "Эскиз60" plane through (-56.55, -30.2, 9.5) normal (0, 0, 1) x (1, 0, 0)
  circle A0 centre (0, 0) radius 0.35 projected
sketch "Эскиз61" plane through (-53.95, -30.2, 9.5) normal (0, 0, 1) x (1, 0, 0)
  circle A0 centre (0, 0) radius 0.35 projected
sketch "Эскиз62" plane through (-51.35, -30.2, 9.5) normal (0, 0, 1) x (1, 0, 0)
  circle A0 centre (0, 0) radius 0.35 projected
sketch "Эскиз63" plane through (-48.75, -30.2, 9.5) normal (0, 0, 1) x (1, 0, 0)
  circle A0 centre (0, 0) radius 0.35 projected
sketch "Эскиз64" plane through (-15.3, -29.7, 9.5) normal (0, 0, 1) x (1, 0, 0)
  circle A0 centre (0, 0) radius 0.35 projected
sketch "Эскиз65" plane through (-15.3, -27.1, 9.5) normal (0, 0, 1) x (1, 0, 0)
  circle A0 centre (0, 0) radius 0.35 projected
sketch "Эскиз66" plane through (-54.4, -1.2, 9.5) normal (0, 0, 1) x (1, 0, 0)
  circle A0 centre (0, 0) radius 0.35 projected
sketch "Эскиз67" plane through (-54.4, 1.4, 9.5) normal (0, 0, 1) x (1, 0, 0)
  circle A0 centre (0, 0) radius 0.35 projected
sketch "Эскиз68" plane through (28.2, 41.9, 9.5) normal (0, 0, 1) x (1, 0, 0)
  circle A0 centre (0, 0) radius 0.35 projected
sketch "Эскиз69" plane through (28.2, 44.5, 9.5) normal (0, 0, 1) x (1, 0, 0)
  circle A0 centre (0, 0) radius 0.35 projected
sketch "Эскиз70" plane through (-18, 61, 9.7) normal (0, 1, 0) x (1, 0, 0)
  line L0 (0, 0) -> (10, 0) projected
  line L1 (-10, 0) -> (-2, 0) projected
  line L2 (-13, 0) -> (-21, 0) projected
  point P0 (18, 9.7)
  point P1 (5, 0)
  point P2 (-6, 0)
  point P3 (-17, 0)
  constraints: 3 midpoint
decal "Маркировка6"
equation "\"d92\" = d88"
equation "\"d93\" = d88"
equation "\"d94\" = d88"
body "Solid1"
